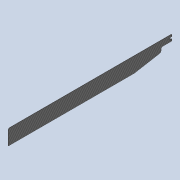
# Autodesk Inventor part: s_carbon_plate5
Saved by Autodesk Inventor 2022 (Build 260153000, 153)
## iProperties
Created: 2021-08-20
Part Number: s_carbon_plate5
Material: CFRP
Document SubType Name: Sheet Metal
Designer: yuta0
Density: 1.43 g/cm^3
Sheet Metal Rule: Default_mm
Appearance: カーボンファイバー
Author: yuta0
Autodesk Inventor part; units mm, degrees
ref_plane "YZ Plane" through (0, 0, 0) normal (1, 0, 0) x (0, 1, 0)
ref_plane "XZ Plane" through (0, 0, 0) normal (0, 1, 0) x (-1, 0, 0)
ref_plane "XY Plane" through (0, 0, 0) normal (0, 0, 1) x (1, 0, 0)
sketch "スケッチ1" plane through (0, 0, 0) normal (1, 0, 0) x (0, 1, 0)
  line L0 (-41, 550) -> (10, 550)
  line L1 (10, 550) -> (10, -10)
  line L2 (10, -10) -> (-41, -10)
  line L3 (-41, -10) -> (-41, 550)
  line L4 (-41, 550) -> (10, -10) construction
  line L5 (10, 550) -> (-41, -10) construction
  point P0 (0, 0)
  dimension "d0" = 51
  dimension "d1" = 560
  dimension "d42" = 10
  dimension "d43" = 10
  measures "d0" distance of L0.start L0.end
  measures "d1" distance of L0.end L1.end
  measures "d42" distance from line of point (0, 0) L2
  measures "d43" distance from line of L1 point (0, 0)
extrude "プレート1" add sketch "スケッチ1" along normal mid plane 1
sketch "スケッチ3" plane through (0.5, 0, 0) normal (1, 0, 0) x (0, 0, -1)
  circle A0 centre (0, 0) radius 6
  line L0 (10, 10) -> (10, -41) projected
  line L1 (-550, 10) -> (10, 10) projected
  point P0 (0, 0)
  point P1 (0, 6)
  point P2 (-6, 0)
  point P3 (0, -6)
  point P4 (6, 0)
  dimension "d13" = 12
  dimension "d14" = 10
  dimension "d15" = 10
  dimension "d18" = 360
  dimension "d44" = 0
  constraints: 1 vertical alignment, 7 other
  measures "d14" distance from line of L0 point (0, 0)
  measures "d15" distance from line of L1 point (0, 0)
  measures "d44" horizontal distance of point (0, 0) point (0, 6)
hole "穴2" at (0.5, 6, 0) at (0.5, 0, 6) at (0.5, -6, 0) at (0.5, 0, -6) direction (-1, 0, 0) diameter 3.2 end through all clearance for "Socket Head Cap Screw" size "M3" standard "Ansi Metric M Profile"
sketch "スケッチ4" plane through (0.5, 0, 0) normal (1, 0, 0) x (0, 0, -1)
  circle A0 centre (0, 0) radius 3.05
  point P0 (0, 0)
  dimension "d27" = 6.1
  constraints: 1 centre point, 1 coincident
  measures "d27" diameter of A0
extrude "押し出し1" cut sketch "スケッチ4" against normal blind 10
sketch "スケッチ5" plane through (0.5, 0, 0) normal (1, 0, 0) x (0, 0, -1)
  line L0 (10, -41) -> (-33.5, -41)
  line L1 (-33.5, -41) -> (-33.5, -10)
  line L2 (-33.5, -10) -> (10, -10)
  line L3 (10, -10) -> (10, -41)
  line L4 (-550, 10) -> (-53.5, 10)
  line L5 (-53.5, 10) -> (-53.5, -12)
  line L6 (-53.5, -12) -> (-550, -12)
  line L7 (-550, -12) -> (-550, 10)
  line L8 (10, -41) -> (-550, -41) projected
  circle A0 centre (0, 0) radius 3.05 projected
  circle A1 centre (0, 0) radius 3.05 projected
  line L9 (0, 3.05) -> (10, 3.05)
  line L10 (0, -3.05) -> (10, -3.05)
  line L11 (10, 10) -> (10, -41) projected
  circle A2 centre (0, 0) radius 10
  circle A3 centre (0, 6) radius 1.6 projected
  circle A4 centre (0, -6) radius 1.6 projected
  line L12 (-550, 10) -> (10, 10) projected
  line L13 (2.95, 10) -> (2.95, -10)
  point P0 (0, 0)
  point P1 (2.95, -3.05)
  point P2 (2.95, 3.05)
  point P3 (2.95, 0.7746)
  point P4 (2.95, -0.7746)
  point P5 (9.5235, -3.05)
  point P6 (0, -10)
  point P7 (0, 10)
  point P8 (9.5235, 3.05)
  point P9 (10, 0)
  point P10 (2.95, -9.555)
  point P11 (2.95, 9.555)
  dimension "d35" = 29
  dimension "d36" = 20
  dimension "d40" = 33.5
  dimension "d41" = 10
  dimension "d45" = 2.95
  constraints: 22 end point, 4 horizontal, 4 parallel, 3 perpendicular, 3 point on line, 3 tangent, 2 point on circle, 1 centre point, 1 coincident
  measures "d35" distance between parallel lines of L8 L6
  measures "d36" distance between parallel lines of L1 L5
  measures "d40" distance from line of A0.centre L1
  measures "d41" distance from line of L2 A0.centre
  measures "d45" distance from line of L13 A3.centre
extrude "押し出し2" cut sketch "スケッチ5" against normal blind 10 contours L0 L1 L2 L3 | L2 L13 A2 L10 L11 | L2 A2 L13 | L10 A2 L11 | L13 L10 A2 | L10 L13 A0 L9 A2 | A2 L9 L11 | L12 L13 A2 | L10 A0 L13 | L9 A2 L13 L12 L11 | L9 L13 A2 | L13 A0 L9 picked at (5.1412, -2.2915)
fillet "コーナーR4" radius 1 4 edges at (0, -3.05, -2.95) (0, 3.05, -2.95) (0, 9.555, -2.95) (0, -9.555, -2.95)
sketch "スケッチ6" plane through (0.5, 0, 0) normal (1, 0, 0) x (0, 0, -1)
  line L0 (-33.5, -41) -> (-550, -41) projected
  line L1 (-33.5, -41) -> (-33.5, -10) projected
  line L2 (-33.5, -25) -> (-124.2405, -41)
  point P0 (0, 0)
  point P1 (-545, -41)
  point P2 (-33.5, -15)
  dimension "d51" = 10
  dimension "d52" = 16
  constraints: 2 end point, 2 point on line
  measures "d51" angle of L0 L2
  measures "d52" distance from line of L0 L2.start
extrude "押し出し3" cut sketch "スケッチ6" against normal blind 10
fillet "コーナーR5" radius 5 2 edges at (0, -25, 33.5) (0, -41, 124.2405)
fillet "コーナーR6" radius 5 2 edges at (0, -10, 33.5) (0, 10, 550)
equation "\"d15\" = d14"
equation "\"d25\" = Thickness"
equation "\"d2\" = Thickness"
equation "\"d43\" = d42"
equation "\"BendRadius\" = Thickness"
equation "\"BendReliefWidth\" = Thickness"
equation "\"BendReliefDepth\" = 0.5 * Thickness"
equation "\"CornerReliefSize\" = 4 * Thickness"
equation "\"MinimumRemnant\" = 2 * Thickness"
equation "\"TransitionRadius\" = BendRadius"
equation "\"JacobiRadiusSize\" = BendRadius"
equation "\"GapSize\" = Thickness"
equation "\"Thickness\" = 1"
